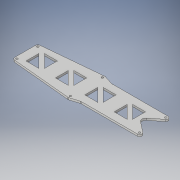
# Autodesk Inventor part: rama_gorna
Saved by Autodesk Inventor 2019 (Build 230136000, 136)
## iProperties
Created: 2020-11-17
Part Number: rama_gorna
Material: Ogólny
Document SubType Name: Modeling
Designer: Karol
Density: 1 g/cm^3
Appearance: Domyślna
Author: Karol
Autodesk Inventor part; units mm, degrees
ref_plane "YZ Plane" through (0, 0, 0) normal (1, 0, 0) x (0, 1, 0)
ref_plane "XZ Plane" through (0, 0, 0) normal (0, 1, 0) x (-1, 0, 0)
ref_plane "XY Plane" through (0, 0, 0) normal (0, 0, 1) x (1, 0, 0)
sketch "Szkic2" plane through (0, 0, 0) normal (0, 1, 0) x (-1, 0, 0)
  circle A0 centre (-88.3883, 88.3883) radius 3 construction
  circle A1 centre (-88.3883, -88.3883) radius 3 construction
  circle A2 centre (88.3883, -88.3883) radius 3 construction
  circle A3 centre (88.3883, 88.3883) radius 3 construction
  circle A4 centre (-88.3883, 96.3883) radius 1.5 construction
  circle A5 centre (-96.3883, 88.3883) radius 1.5 construction
  circle A6 centre (-88.3883, 80.3883) radius 1.5 construction
  circle A7 centre (-80.3883, 88.3883) radius 1.5 construction
  circle A8 centre (-96.3883, -88.3883) radius 1.5 construction
  circle A9 centre (-88.3883, -96.3883) radius 1.5 construction
  circle A10 centre (-88.3883, -80.3883) radius 1.5 construction
  circle A11 centre (-80.3883, -88.3883) radius 1.5 construction
  circle A12 centre (88.3883, -96.3883) radius 1.5 construction
  circle A13 centre (96.3883, -88.3883) radius 1.5 construction
  circle A14 centre (80.3883, -88.3883) radius 1.5 construction
  circle A15 centre (88.3883, -80.3883) radius 1.5 construction
  circle A16 centre (96.3883, 88.3883) radius 1.5 construction
  circle A17 centre (88.3883, 96.3883) radius 1.5 construction
  circle A18 centre (88.3883, 80.3883) radius 1.5 construction
  circle A19 centre (80.3883, 88.3883) radius 1.5 construction
  line L0 (82.7315, 75.6604) -> (89.8026, 75.6604) construction
  line L1 (89.8026, 75.6604) -> (101.1163, 86.9741) construction
  line L2 (101.1163, 86.9741) -> (101.1163, 94.0452) construction
  line L3 (101.1163, 94.0452) -> (94.0452, 101.1163) construction
  line L4 (94.0452, 101.1163) -> (86.9741, 101.1163) construction
  line L5 (86.9741, 101.1163) -> (75.6604, 89.8026) construction
  line L6 (75.6604, 89.8026) -> (75.6604, 82.7315) construction
  line L7 (75.6604, 82.7315) -> (23.3934, 30.4645) construction
  arc A20 (19.8579, 29) -> (23.3934, 30.4645) centre (19.8579, 34) ccw construction
  line L8 (19.8579, 29) -> (-19.8579, 29) construction
  arc A21 (-23.3934, 30.4645) -> (-19.8579, 29) centre (-19.8579, 34) ccw construction
  line L9 (-23.3934, 30.4645) -> (-75.6604, 82.7315) construction
  line L10 (-75.6604, 82.7315) -> (-75.6604, 89.8026) construction
  line L11 (-75.6604, 89.8026) -> (-86.9741, 101.1163) construction
  line L12 (-86.9741, 101.1163) -> (-94.0452, 101.1163) construction
  line L13 (-94.0452, 101.1163) -> (-101.1163, 94.0452) construction
  line L14 (-101.1163, 94.0452) -> (-101.1163, 86.9741) construction
  line L15 (-101.1163, 86.9741) -> (-89.8026, 75.6604) construction
  line L16 (-89.8026, 75.6604) -> (-82.7315, 75.6604) construction
  line L17 (-82.7315, 75.6604) -> (-44.6066, 37.5355) construction
  arc A22 (-48.1421, 29) -> (-44.6066, 37.5355) centre (-48.1421, 34) ccw construction
  line L18 (-48.1421, 29) -> (-92.6893, 29) construction
  arc A23 (-92.6893, 29) -> (-94.2344, 28.7553) centre (-92.6893, 24) ccw construction
  line L19 (-94.2344, 28.7553) -> (-106.5451, 24.7553) construction
  arc A24 (-106.5451, 24.7553) -> (-110, 20) centre (-105, 20) ccw construction
  line L20 (-110, 20) -> (-110, -20) construction
  arc A25 (-110, -20) -> (-106.5451, -24.7553) centre (-105, -20) ccw construction
  line L21 (-106.5451, -24.7553) -> (-94.2344, -28.7553) construction
  arc A26 (-94.2344, -28.7553) -> (-92.6893, -29) centre (-92.6893, -24) ccw construction
  line L22 (-92.6893, -29) -> (-48.1421, -29) construction
  arc A27 (-44.6066, -37.5355) -> (-48.1421, -29) centre (-48.1421, -34) ccw construction
  line L23 (-44.6066, -37.5355) -> (-82.7315, -75.6604) construction
  line L24 (-82.7315, -75.6604) -> (-89.8026, -75.6604) construction
  line L25 (-89.8026, -75.6604) -> (-101.1163, -86.9741) construction
  line L26 (-101.1163, -86.9741) -> (-101.1163, -94.0452) construction
  line L27 (-101.1163, -94.0452) -> (-94.0452, -101.1163) construction
  line L28 (-94.0452, -101.1163) -> (-86.9741, -101.1163) construction
  line L29 (-86.9741, -101.1163) -> (-75.6604, -89.8026) construction
  line L30 (-75.6604, -89.8026) -> (-75.6604, -82.7315) construction
  line L31 (-75.6604, -82.7315) -> (-23.3934, -30.4645) construction
  arc A28 (-19.8579, -29) -> (-23.3934, -30.4645) centre (-19.8579, -34) ccw construction
  line L32 (-19.8579, -29) -> (19.8579, -29) construction
  arc A29 (23.3934, -30.4645) -> (19.8579, -29) centre (19.8579, -34) ccw construction
  line L33 (23.3934, -30.4645) -> (75.6604, -82.7315) construction
  line L34 (75.6604, -82.7315) -> (75.6604, -89.8026) construction
  line L35 (75.6604, -89.8026) -> (86.9741, -101.1163) construction
  line L36 (86.9741, -101.1163) -> (94.0452, -101.1163) construction
  line L37 (94.0452, -101.1163) -> (101.1163, -94.0452) construction
  line L38 (101.1163, -94.0452) -> (101.1163, -86.9741) construction
  line L39 (101.1163, -86.9741) -> (89.8026, -75.6604) construction
  line L40 (89.8026, -75.6604) -> (82.7315, -75.6604) construction
  line L41 (82.7315, -75.6604) -> (44.6066, -37.5355) construction
  arc A30 (48.1421, -29) -> (44.6066, -37.5355) centre (48.1421, -34) ccw construction
  line L42 (48.1421, -29) -> (73.1421, -29) construction
  arc A31 (73.1421, -29) -> (77.0275, -28.2143) centre (73.1421, -19) ccw construction
  line L43 (77.0275, -28.2143) -> (88.8853, -23.2143) construction
  arc A32 (88.8853, -23.2143) -> (95, -14) centre (85, -14) ccw construction
  line L44 (95, -14) -> (95, 14) construction
  arc A33 (95, 14) -> (88.8853, 23.2143) centre (85, 14) ccw construction
  line L45 (88.8853, 23.2143) -> (77.0275, 28.2143) construction
  arc A34 (77.0275, 28.2143) -> (73.1421, 29) centre (73.1421, 19) ccw construction
  line L46 (73.1421, 29) -> (48.1421, 29) construction
  arc A35 (44.6066, 37.5355) -> (48.1421, 29) centre (48.1421, 34) ccw construction
  line L47 (44.6066, 37.5355) -> (82.7315, 75.6604) construction
  circle A36 centre (-3.5, 24.5) radius 1.5
  circle A37 centre (87, 16) radius 1.5
  circle A38 centre (-105, 20) radius 1.5
  line L48 (0, 0) -> (95, 0) construction
  line L49 (0, 0) -> (0, 60.6938) construction
  circle A39 centre (87, -16) radius 1.5
  circle A40 centre (-105, -20) radius 1.5
  circle A41 centre (-3.5, -24.5) radius 1.5
  line L50 (223.398, 0) -> (223.398, -75.6604) construction
  line L51 (223.398, -75.6604) -> (321.3499, 0) construction
  line L52 (321.3499, 0) -> (228.4095, 80.3883) construction
  line L53 (228.4095, 80.3883) -> (228.4095, 19.0873) construction
  line L54 (228.4095, 19.0873) -> (177.4792, 19.0873) construction
  line L55 (177.4792, 19.0873) -> (177.4792, 0) construction
  line L56 (177.4792, 0) -> (223.398, 0) construction
  circle A42 centre (-88.3883, 88.3883) radius 63.5 construction
  circle A43 centre (88.3883, 88.3883) radius 63.5 construction
  arc A44 (-105, 23.5) -> (-107.1496, 17.2379) centre (-105, 20) ccw
  line L57 (-91.0842, 4.735) -> (-107.1496, 17.2379)
  line L58 (-105, 23.5) -> (-19.5, 23.5)
  arc A45 (90.5, 16) -> (87.3273, 19.4847) centre (87, 16) ccw
  line L59 (90.5, 16) -> (90.5, 0)
  arc A46 (-19.5, 23.5) -> (-17.729, 23.7673) centre (-19.5, 29.5) ccw
  arc A47 (-3.1727, 27.9847) -> (-4.5331, 27.8441) centre (-3.5, 24.5) ccw
  line L60 (-17.729, 23.7673) -> (-4.5331, 27.8441)
  line L61 (-3.1727, 27.9847) -> (87.3273, 19.4847)
  arc A48 (-107.1496, -17.2379) -> (-105, -23.5) centre (-105, -20) ccw
  line L62 (-91.0842, -4.735) -> (-107.1496, -17.2379)
  arc A49 (87.3273, -19.4847) -> (90.5, -16) centre (87, -16) ccw
  line L63 (90.5, -16) -> (90.5, 0)
  arc A50 (-4.5331, -27.8441) -> (-3.1727, -27.9847) centre (-3.5, -24.5) ccw
  line L64 (-3.1727, -27.9847) -> (87.3273, -19.4847)
  arc A51 (-91.0842, -4.735) -> (-91.0842, 4.735) centre (-94.7692, 0) ccw
  line L65 (-85, 15) -> (-55, 15) construction
  line L66 (-55, 15) -> (-55, -15) construction
  line L67 (-55, -15) -> (-85, -15) construction
  line L68 (-85, -15) -> (-85, 15) construction
  line L69 (-85, 15) -> (-55, -15) construction
  line L70 (-55, 15) -> (-85, -15) construction
  line L71 (-58, -7.7574) -> (-58, 12)
  line L72 (-58, 12) -> (-77.7574, 12)
  line L73 (-77.7574, 12) -> (-58, -7.7574)
  line L74 (-62.2426, -12) -> (-82, -12)
  line L75 (-82, -12) -> (-82, 7.7574)
  line L76 (-82, 7.7574) -> (-62.2426, -12)
  line L77 (-13, 12) -> (-32.7574, 12)
  line L78 (-13, -7.7574) -> (-13, 12)
  line L79 (-32.7574, 12) -> (-13, -7.7574)
  line L80 (-37, 7.7574) -> (-17.2426, -12)
  line L81 (-37, -12) -> (-37, 7.7574)
  line L82 (-17.2426, -12) -> (-37, -12)
  line L83 (32, 12) -> (12.2426, 12)
  line L84 (32, -7.7574) -> (32, 12)
  line L85 (12.2426, 12) -> (32, -7.7574)
  line L86 (8, 7.7574) -> (27.7574, -12)
  line L87 (8, -12) -> (8, 7.7574)
  line L88 (27.7574, -12) -> (8, -12)
  line L89 (77, 12) -> (57.2426, 12)
  line L90 (77, -7.7574) -> (77, 12)
  line L91 (57.2426, 12) -> (77, -7.7574)
  line L92 (53, 7.7574) -> (72.7574, -12)
  line L93 (53, -12) -> (53, 7.7574)
  line L94 (72.7574, -12) -> (53, -12)
  line L95 (-105, -23.5) -> (-19.5, -23.5)
  arc A52 (-17.729, -23.7673) -> (-19.5, -23.5) centre (-19.5, -29.5) ccw
  line L96 (-17.729, -23.7673) -> (-4.5331, -27.8441)
  point P0 (-70, 0)
  point P1 (-60, 0)
  point P2 (47.066, 0)
  point P3 (-85, 0)
  point P4 (-19.1898, 23.5)
  point P5 (-70, 0)
  dimension "d26" = 3
  dimension "d27" = 20
  dimension "d28" = 16
  dimension "d29" = 8
  dimension "d40" = 110
  dimension "d41" = 29
  dimension "d42" = 95
  dimension "d43" = 24.5
  dimension "d44" = 3.5
  dimension "d45" = 5
  dimension "d46" = 127
  dimension "d47" = 127
  dimension "d48" = 7
  dimension "d49" = 7
  dimension "d50" = 25
  dimension "d51" = 6
  dimension "d52" = 7
  dimension "d53" = 16
  dimension "d54" = 6
  dimension "d55" = 30
  dimension "d56" = 30
  dimension "d57" = 70
  dimension "d58" = 3
  dimension "d61" = 45
  constraints: 194 end point, 54 point on circle, 53 centre point, 19 symmetric about line, 10 tangent, 7 coincident, 7 point on line, 6 perpendicular, 4 horizontal, 4 midpoint, 3 horizontal alignment, 3 parallel, 2 equal radius, 2 vertical, 45 other
  measures "d26" diameter of A37
  measures "d27" distance from line of L48 A38.centre
  measures "d28" distance from line of A37.centre L48
  measures "d29" distance from line of L44 A37.centre
  measures "d40" distance between parallel lines of L20 L49
  measures "d41" distance between parallel lines of L48 L18
  measures "d42" distance between parallel lines of L44 L49
  measures "d43" distance from line of L48 A36.centre
  measures "d44" distance from line of L49 A36.centre
  measures "d45" distance from line of L20 A38.centre
  measures "d46" diameter of A42
  measures "d47" diameter of A43
  measures "d48" diameter of A44
  measures "d49" diameter of A45
  measures "d50" distance from line of L20 point (-85, 0)
  measures "d51" radius of A46
  measures "d52" diameter of A47
  measures "d53" horizontal distance of A46.centre A36.centre
  measures "d54" radius of A51
  measures "d55" distance of L65.end L66.end
  measures "d56" distance of L65.start L65.end
  measures "d57" distance of point (0, 0) point (-70, 0)
  measures "d58" distance between parallel lines of L69 L73
  measures "d61" distance of L71.end L77.start
extrude "Wyciągnięcie proste1" add sketch "Szkic2" along normal blind 3
